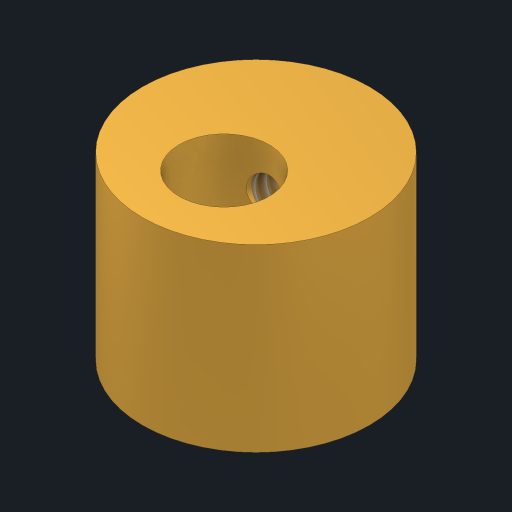
# Autodesk Inventor part: Capper Gate Bushing
Saved by Autodesk Inventor 2023.1 (Build 271208000, 208)
## iProperties
Created: 2023-05-23
Part Number: Capper Gate Bushing
Material: Brass, Soft Yellow
Document SubType Name: Modeling
Designer: Jarrett
Density: 8.47 g/cm^3
Appearance: Brass - Satin
Author: Jarrett
Autodesk Inventor part; units mm, degrees
note: some values were not read from the file. Chosen so that the rebuilt part matches the saved one: direction of "Hole1".
ref_plane "YZ Plane" through (0, 0, 0) normal (1, 0, 0) x (0, 1, 0)
ref_plane "XZ Plane" through (0, 0, 0) normal (0, 1, 0) x (-1, 0, 0)
sketch "Sketch1" plane through (0, 0, 0) normal (0, 1, 0) x (-1, 0, 0)
  circle A0 centre (0, 0) radius 3.175
  circle A1 centre (0, -2.25) radius 8
  line L0 (0, -2.25) -> (0, 0) construction
  circle A2 centre (0, 0) radius 4.7625 construction
  dimension "d5" = 6.35
  dimension "d6" = 2.25
  dimension "d9" = 9.525
  dimension "d11" = 16
  constraints: 3 centre point, 2 coincident, 2 end point, 1 vertical
  measures "d5" diameter of A0
  measures "d6" distance of L0.start L0.end
  measures "d9" diameter of A2
  measures "d11" diameter of A1
extrude "Extrusion1" add sketch "Sketch1" along normal blind 12.7
ref_plane "Work Plane1" through (0, 0, -10.25) normal (0, 0, 1) x (1, 0, 0)
sketch "Sketch2" plane through (0, 0, -10.25) normal (0, 0, 1) x (1, 0, 0)
  circle A0 centre (0, 3.175) radius 1.7272
  line L0 (0, -2.54) -> (0, 15.24) construction
  circle A1 centre (0, 9.525) radius 1.7272
  line L1 (8, 0) -> (-8, 0) projected
  line L2 (8, 12.7) -> (-8, 12.7) projected
  point P0 (0, 0)
  dimension "d14" = 3.4544
  dimension "d15" = 3.4544
  dimension "d16" = 3.175
  dimension "d17" = 3.175
  constraints: 2 centre point, 2 coincident, 2 point on line
  measures "d14" diameter of A0
  measures "d15" diameter of A1
  measures "d16" distance from line of A0.centre L1
  measures "d17" distance from line of L2 A1.centre
hole "Hole1" at (0, 3.175, -10.25) at (0, 9.525, -10.25) direction (0, 0, 1) diameter 2.6416 end up to surface thread size "6-32 UNC" class "2B" standard "ANSI Unified Screw Threads"
equation "\"d15\" = d14"
equation "\"d16\" = 0.25 * d12"
equation "\"d17\" = 0.25 * d12"
equation "\"d12\" = 12.7"
body "Solid1"
